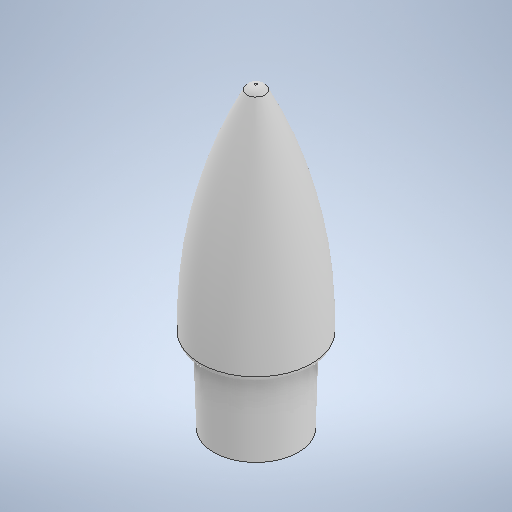
# Autodesk Inventor part: noseconefairing
Saved by Autodesk Inventor 2025.2 (Build 292293000, 293)
## iProperties
Created: 2024-11-15
Part Number: noseconefairing
Material: Generic
Document SubType Name: Sheet Metal
Designer: jadba
Density: 1 g/cm^3
Sheet Metal Rule: Default_mm
Appearance: Default
Author: jadba
Autodesk Inventor part; units mm, degrees
ref_plane "YZ Plane" through (0, 0, 0) normal (1, 0, 0) x (0, 1, 0)
ref_plane "XZ Plane" through (0, 0, 0) normal (0, 1, 0) x (-1, 0, 0)
ref_plane "XY Plane" through (0, 0, 0) normal (0, 0, 1) x (1, 0, 0)
sketch "Sketch1" plane through (0, 0, 0) normal (0, 0, 1) x (1, 0, 0)
  line L0 (0, 0) -> (-19.2, 0)
  line L1 (-19.2, 0) -> (-20.2, 35)
  line L2 (-20.2, 35) -> (-25.2, 35)
  arc A0 (-3, 135) -> (-25.2, 35) centre (174.6359, 43.1006) ccw
  line L3 (-3, 135) -> (0, 135)
  line L4 (0, 135) -> (0, 0)
  dimension "d0" = 19.2
  dimension "d1" = 35
  dimension "d2" = 1
  dimension "d3" = 5
  dimension "d4" = 200
  dimension "d5" = 100
  dimension "d6" = 3
  constraints: 10 end point, 3 horizontal, 2 point on circle, 1 centre point, 1 vertical
  measures "d0" distance of L0.start L0.end
  measures "d1" vertical distance of L0.end L1.end
  measures "d2" horizontal distance of L0.end L1.end
  measures "d3" distance of L1.end L2.end
  measures "d4" radius of A0
  measures "d5" vertical distance of L1.end L3.start
  measures "d6" horizontal distance of L0.start L3.start
revolve "Revolution1" add sketch "Sketch1" angle 360 about axis through (0, 135, 0) along (0, -1, 0)
fillet "Fillet1" radius 4 1 edges at (3, 135, 0)
fillet "Fillet2" radius 3 1 edges at (25.2, 35, 0)
equation "\"BendRadius\" = Thickness"
equation "\"BendReliefWidth\" = Thickness"
equation "\"BendReliefDepth\" = 0.5 * Thickness"
equation "\"CornerReliefSize\" = 4 * Thickness"
equation "\"MinimumRemnant\" = 2 * Thickness"
equation "\"TransitionRadius\" = BendRadius"
equation "\"JacobiRadiusSize\" = BendRadius"
equation "\"GapSize\" = Thickness"
equation "\"Thickness\" = 0.5"
body "Solid1"
